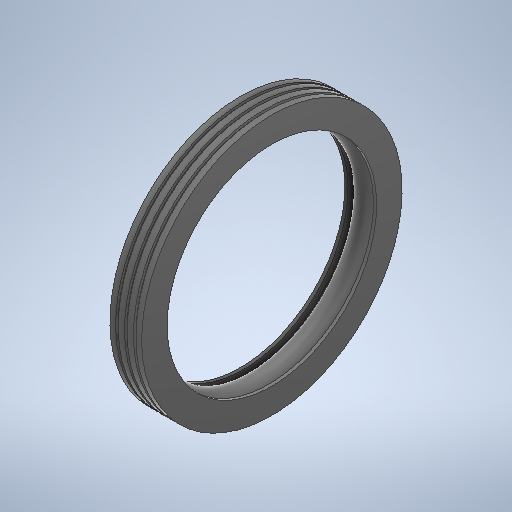
# Autodesk Inventor part: TPU Tire
Saved by Autodesk Inventor 2025.2 (Build 292293000, 293)
## iProperties
Created: 2025-01-18
Part Number: TPU Tire
Material: Generic
Document SubType Name: Modeling
Designer: mtidd
Density: 1 g/cm^3
Appearance: Default
Author: mtidd
Autodesk Inventor part; units mm, degrees
ref_plane "YZ Plane" through (0, 0, 0) normal (1, 0, 0) x (0, 1, 0)
ref_plane "XZ Plane" through (0, 0, 0) normal (0, 1, 0) x (-1, 0, 0)
ref_plane "XY Plane" through (0, 0, 0) normal (0, 0, 1) x (1, 0, 0)
sketch "Sketch3" plane through (0, 0, 0) normal (0, 0, 1) x (1, 0, 0)
  arc A0 (-7.5, 7.5) -> (7.5, 7.5) centre (0, 7.5) ccw
  line L0 (-7.5, 7.5) -> (-10, 7.5)
  line L1 (0, -80) -> (50, -80)
  line L2 (0, -80) -> (50, -80) construction
  line L3 (-10, 7.5) -> (10, 7.5)
  line L4 (10, 7.5) -> (10, 22.5)
  line L5 (10, 22.5) -> (-10, 22.5)
  line L6 (-10, 22.5) -> (-10, 7.5)
  line L7 (10, 22.5) -> (12.5, 22.5)
  line L8 (12.5, 22.5) -> (12.5, 2.5)
  line L9 (12.5, 2.5) -> (10, 2.5)
  line L10 (10, 2.5) -> (10, 22.5)
  line L11 (-10, 22.5) -> (-12.5, 22.5)
  line L12 (-12.5, 22.5) -> (-12.5, 2.5)
  line L13 (-12.5, 2.5) -> (-10, 2.5)
  line L14 (-10, 2.5) -> (-10, 22.5)
  line L15 (-10, 22.5) -> (-8, 22.5)
  line L16 (-10, 22.5) -> (-8, 22.5) construction
  line L17 (-8, 22.5) -> (-8, 20.5)
  line L18 (-8, 20.5) -> (-6, 20.5)
  line L19 (-6, 20.5) -> (-6, 22.5)
  line L20 (-1, 22.5) -> (1, 22.5)
  line L21 (1, 22.5) -> (1, 20.5)
  line L22 (1, 20.5) -> (-1, 20.5)
  line L23 (-1, 20.5) -> (-1, 22.5)
  line L24 (6, 22.5) -> (8, 22.5)
  line L25 (8, 22.5) -> (8, 20.5)
  line L26 (8, 20.5) -> (6, 20.5)
  line L27 (6, 20.5) -> (6, 22.5)
  point P0 (0, 0)
  point P1 (7.5, 7.5)
  point P2 (1, 22.5)
  dimension "d19" = 2.5
  dimension "d34" = 0
  dimension "d35" = 20
  dimension "d36" = 15
  dimension "d37" = 2.5
  dimension "d38" = 20
  dimension "d39" = 2.5
  dimension "d40" = 20
  dimension "d41" = 2
  dimension "d42" = 0
  dimension "d43" = 2
  dimension "d44" = 2
  dimension "d45" = 2
  dimension "d46" = 2
  dimension "d47" = 2
  dimension "d48" = 2
  dimension "d49" = 5
  dimension "d50" = 5
  constraints: 56 end point, 10 parallel, 8 horizontal, 8 perpendicular, 3 collinear, 3 point on circle, 3 point on line, 1 centre point
  measures "d19" distance of L0.start L0.end
  measures "d34" distance between parallel lines of L1 L2
  measures "d35" distance of L5.end L4.end
  measures "d36" distance of L4.end L3.end
  measures "d37" distance of L8.end L9.end
  measures "d38" distance of L7.end L8.end
  measures "d39" distance of L13.end L12.end
  measures "d40" distance of L12.end L11.end
  measures "d41" distance of L5.end L15.end
  measures "d42" distance between parallel lines of L15 L16
  measures "d43" distance of L15.end L17.end
  measures "d44" distance of L17.end L18.end
  measures "d45" distance of L21.end L22.end
  measures "d46" distance of L20.end L21.end
  measures "d47" distance of L25.end L26.end
  measures "d48" distance of L24.end L25.end
  measures "d49" distance between parallel lines of L23 L19
  measures "d50" distance between parallel lines of L27 L21
revolve "Revolution2" add sketch "Sketch3" angle 360 about axis through (0, -80, 0) along (1, 0, 0) contours L3 A0 | L0 L6 L5 L17 L18 L19 L23 L22 L21 L27 L26 L25 L4 L3 | L14 L13 L12 L11 L6 | L4 L7 L8 L9 L10
body "Solid2"
